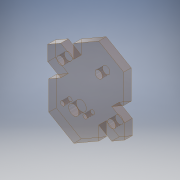
# Autodesk Inventor part: Dribbler Plate
Saved by Autodesk Inventor 2017 (Build 210142000, 142)
## iProperties
Created: 2017-04-14
Part Number: Dribbler Plate
Material: Polycarbonate, Smoke
Document SubType Name: Modeling
Designer: yella
Density: 1.2 g/cm^3
Appearance: Polycarbonate - Smoked
Author: yella
Autodesk Inventor part; units mm, degrees
ref_plane "YZ Plane" through (0, 0, 0) normal (1, 0, 0) x (0, 1, 0)
ref_plane "XZ Plane" through (0, 0, 0) normal (0, 1, 0) x (-1, 0, 0)
ref_plane "XY Plane" through (0, 0, 0) normal (0, 0, 1) x (1, 0, 0)
sketch "Sketch1" plane through (0, 0, 0) normal (0, 1, 0) x (-1, 0, 0)
  circle A0 centre (0, 0) radius 2.05
  line L0 (0, 0) -> (-4.5, 0)
  line L1 (0, 0) -> (4.5, 0)
  circle A1 centre (-4.5, 0) radius 0.85
  circle A2 centre (4.5, 0) radius 0.85
  line L2 (0, 0) -> (-5, 8.6603)
  line L3 (0, 0) -> (10, 0) construction
  line L4 (0, 11.547) -> (10, 5.7735)
  line L5 (10, 5.7735) -> (10, -5.7735)
  line L6 (10, -5.7735) -> (0, -11.547)
  line L7 (0, -11.547) -> (-10, -5.7735)
  line L8 (-10, -5.7735) -> (-10, 5.7735)
  line L9 (-10, 5.7735) -> (0, 11.547)
  line L10 (-5, 8.6603) -> (-10, 17.3205)
  line L11 (-10, 5.7735) -> (-20, 11.547)
  line L12 (-20, 11.547) -> (-20, 23.094)
  line L13 (-20, 23.094) -> (-10, 28.8675)
  line L14 (-10, 28.8675) -> (0, 23.094)
  line L15 (0, 23.094) -> (0, 11.547)
  line L16 (0, 11.547) -> (-10, 5.7735)
  circle A3 centre (-10, 17.3205) radius 1.5
  circle A4 centre (-15.1962, 2.7735) radius 1.6
  circle A5 centre (5.1962, 14.547) radius 1.6
  line L17 (0, 11.547) -> (5.1962, 14.547)
  line L18 (-10, 5.7735) -> (-15.1962, 2.7735)
  line L19 (-10, 5.7735) -> (-10, -0.2265)
  line L20 (-10, -0.2265) -> (-15.1962, -3.2265)
  line L21 (-15.1962, -3.2265) -> (-20.3923, -0.2265)
  line L22 (-20.3923, -0.2265) -> (-20.3923, 5.7735)
  line L23 (-20.3923, 5.7735) -> (-15.1962, 8.7735)
  line L24 (-15.1962, 8.7735) -> (-10, 5.7735)
  line L25 (0, 11.547) -> (0, 17.547)
  line L26 (0, 17.547) -> (5.1962, 20.547)
  line L27 (5.1962, 20.547) -> (10.3923, 17.547)
  line L28 (10.3923, 17.547) -> (10.3923, 11.547)
  line L29 (10.3923, 11.547) -> (5.1962, 8.547)
  line L30 (5.1962, 8.547) -> (0, 11.547)
  dimension "d0" = 4.1
  dimension "d16" = 4.5
  dimension "d17" = 4.5
  dimension "d18" = 1.7
  dimension "d19" = 1.7
  dimension "d20" = 10
  dimension "d21" = 120
  dimension "d22" = 10
  dimension "d23" = 3
  dimension "d26" = 3.2
  dimension "d27" = 3.2
  dimension "d28" = 6
  dimension "d29" = 6
  constraints: 62 end point, 12 coincident, 6 centre point, 3 horizontal, 1 equal length, 52 other
  measures "d0" diameter of A0
  measures "d16" distance of L0.start L0.end
  measures "d17" distance of L0.start L1.end
  measures "d18" diameter of A1
  measures "d19" diameter of A2
  measures "d20" distance of L0.start L2.end
  measures "d21" angle of L3 L2
  measures "d22" distance of L2.end L10.end
  measures "d23" diameter of A3
  measures "d26" diameter of A4
  measures "d27" diameter of A5
  measures "d28" distance of L15.end L17.end
  measures "d29" distance of L8.end L18.end
extrude "Extrusion1" add sketch "Sketch1" along normal blind 3
body "Solid1"
